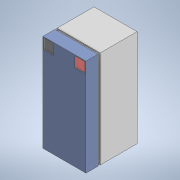
# Autodesk Inventor part: 1.4AH SLAB
Saved by Autodesk Inventor 2020 (Build 240168000, 168)
## iProperties
Created: 2020-04-08
Part Number: 1.4AH SLAB
Material: Generic
Document SubType Name: Modeling
Designer: angusaitken
Density: 1 g/cm^3
Appearance: Default
Author: angusaitken
Autodesk Inventor part; units mm, degrees
ref_plane "YZ Plane" through (0, 0, 0) normal (1, 0, 0) x (0, 1, 0)
ref_plane "XZ Plane" through (0, 0, 0) normal (0, 1, 0) x (-1, 0, 0)
ref_plane "XY Plane" through (0, 0, 0) normal (0, 0, 1) x (1, 0, 0)
sketch "Sketch1" plane through (0, 0, 0) normal (0, 1, 0) x (-1, 0, 0)
  line L0 (0, 0) -> (-40, 0)
  line L1 (-40, 0) -> (-40, -50)
  line L2 (-40, -50) -> (0, -50)
  line L3 (0, -50) -> (0, 0)
  dimension "d0" = 40
  dimension "d1" = 50
  constraints: 8 end point, 2 parallel, 1 horizontal, 1 perpendicular
  measures "d0" distance of L2.end L1.end
  measures "d1" distance of L1.end L0.end
extrude "Extrusion1" add sketch "Sketch1" along normal blind 100
move faces "Move1" translate (0, 0, -13) faces at (13.3333, 33.3333, 0)
sketch "Sketch2" plane through (0, 0, -13) normal (0, 0, 1) x (1, 0, 0)
  line L0 (0, 0) -> (40, 0) projected
  line L1 (40, 0) -> (40, 100) projected
  line L2 (0, 100) -> (40, 100) projected
  line L3 (0, 0) -> (0, 100) projected
  line L4 (39, 99) -> (39, 1)
  line L5 (39, 1) -> (1, 1)
  line L6 (1, 1) -> (1, 99)
  line L7 (1, 99) -> (39, 99)
  dimension "d7" = 1
  constraints: 8 end point, 3 other
  measures "d7" distance between parallel lines of L2 L7
extrude "Extrusion2" add sketch "Sketch2" along normal blind 2 contours L4 L5 L6 L7
sketch "Sketch3" plane through (0, 0, -11) normal (0, 0, 1) x (1, 0, 0)
  line L0 (0, 100) -> (40, 100) projected
  line L1 (0, 0) -> (0, 100) projected
  line L2 (40, 0) -> (40, 100) projected
  line L3 (0, 0) -> (40, 0) projected
extrude "Extrusion3" add sketch "Sketch3" along normal blind 12
move faces "Move2" translate (3, 0, 0) faces at (40, 66.6667, -37.6667) (39, 33.6667, -12.3333) (40, 33.3333, -7)
move faces "Move3" translate (0, -3, 0) faces at (28.6667, 100, -25.3333) (14.6667, 99, -11.6667) (14.3333, 100, -3)
sketch "Sketch4" plane through (0, 0, 1) normal (0, 0, 1) x (1, 0, 0)
  line L0 (0, 97) -> (0, 0) projected
  line L1 (0, 0) -> (43, 0) projected
  line L2 (43, 0) -> (43, 97) projected
  line L3 (43, 97) -> (0, 97) projected
  line L4 (1, 96) -> (1, 1)
  line L5 (1, 1) -> (42, 1)
  line L6 (42, 1) -> (42, 96)
  line L7 (42, 96) -> (1, 96)
  line L8 (1, 96) -> (42, 96) projected
  line L9 (1, 96) -> (11, 96)
  line L10 (11, 96) -> (11, 86)
  line L11 (11, 86) -> (1, 86)
  line L12 (1, 86) -> (1, 96)
  line L13 (42, 96) -> (32, 96)
  line L14 (32, 96) -> (32, 86)
  line L15 (32, 86) -> (42, 86)
  line L16 (42, 86) -> (42, 96)
  dimension "d18" = 1
  dimension "d19" = 10
  dimension "d20" = 10
  dimension "d21" = 10
  dimension "d22" = 10
  constraints: 24 end point, 4 parallel, 2 perpendicular, 3 other
  measures "d18" distance between parallel lines of L3 L7
  measures "d19" distance of L10.end L11.end
  measures "d20" distance of L9.end L10.end
  measures "d21" distance of L15.end L14.end
  measures "d22" distance of L13.end L14.end
extrude "Extrusion4" cut sketch "Sketch4" against normal blind 0.5 contours L7 L10 L11 L4 | L7 L6 L15 L14
equation "\"d22\" = d20"
body "Solid1"
